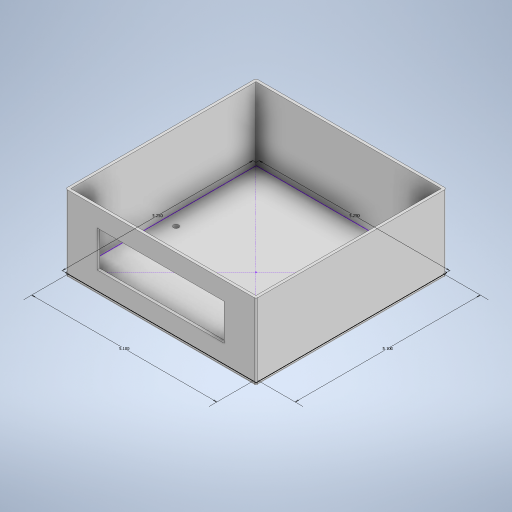
# Autodesk Inventor part: TC720 box
Saved by Autodesk Inventor 2024.1 (Build 281209000, 209)
## iProperties
Created: 2024-09-06
Part Number: TC720 box
Material: Generic
Document SubType Name: Modeling
Designer: pab2
Density: 1 g/cm^3
Appearance: Default
Author: pab2
Autodesk Inventor part; units mm, degrees
ref_plane "YZ Plane" through (0, 0, 0) normal (1, 0, 0) x (0, 1, 0)
ref_plane "XZ Plane" through (0, 0, 0) normal (0, 1, 0) x (-1, 0, 0)
ref_plane "XY Plane" through (0, 0, 0) normal (0, 0, 1) x (1, 0, 0)
sketch "Sketch1" plane through (0, 0, 0) normal (0, 1, 0) x (-1, 0, 0)
  line L0 (0, 0) -> (133.35, 0)
  line L1 (133.35, 0) -> (133.35, -133.35)
  line L2 (133.35, -133.35) -> (0, -133.35)
  line L3 (0, -133.35) -> (0, 0)
  line L4 (131.445, -131.445) -> (1.905, -131.445)
  line L5 (1.905, -131.445) -> (1.905, -1.905)
  line L6 (1.905, -1.905) -> (131.445, -1.905)
  line L7 (131.445, -1.905) -> (131.445, -131.445)
  line L8 (131.445, -131.445) -> (1.905, -1.905) construction
  line L9 (1.905, -131.445) -> (131.445, -1.905) construction
  point P0 (66.675, -66.675)
  dimension "d0" = 133.35
  dimension "d1" = 133.35
  dimension "d2" = 129.54
  dimension "d3" = 129.54
  constraints: 20 end point, 4 parallel, 2 horizontal, 2 midpoint, 2 perpendicular
  measures "d0" distance of L1.end L2.end
  measures "d1" distance of L0.end L1.end
  measures "d2" distance of L5.end L6.end
  measures "d3" distance of L4.end L5.end
extrude "Extrusion1" add sketch "Sketch1" along normal blind 50.8
extrude "Extrusion2" add sketch "Sketch1" against normal blind 2.54 contours L0 L1 L2 L3 | L4 L5 L6 L7
fillet "Fillet1" radius 1.27 8 edges at (0, 24.13, 0) (0, -2.54, -66.675) (-66.675, -2.54, 0) (0, 24.13, -133.35) (-66.675, -2.54, -133.35) (-133.35, 24.13, -133.35) (-133.35, -2.54, -66.675) (-133.35, 24.13, 0)
sketch "Sketch2" plane through (0, 0, 0) normal (0, 1, 0) x (1, 0, 0)
  line L0 (-131.445, 1.905) -> (-131.445, 131.445) projected
  line L1 (-1.905, 1.905) -> (-131.445, 1.905) projected
  line L2 (-1.905, 131.445) -> (-1.905, 1.905) projected
  line L3 (-131.445, 131.445) -> (-1.905, 131.445) projected
  line L4 (-66.675, 66.675) -> (-10.795, 66.675)
  line L5 (-66.675, 66.675) -> (-10.795, 66.675) construction
  line L6 (-10.795, 66.675) -> (-122.555, 66.675)
  point P0 (0, 0)
  dimension "d9" = 55.88
  dimension "d10" = 0
  dimension "d11" = 111.76
  constraints: 6 end point, 2 horizontal, 1 collinear, 1 point on line
  measures "d9" distance of L4.start L4.end
  measures "d10" distance between parallel lines of L4 L5
  measures "d11" distance of L4.end L6.end
hole "Hole1" at (-10.795, 0, -66.675) at (-122.555, 0, -66.675) direction (0, -1, 0) diameter 3.6576 end through all
sketch "Sketch3" plane through (-132.08, -1.27, 0) normal (0, 0, 1) x (1, 0, 0)
  line L0 (130.175, 1.27) -> (0.635, 1.27) projected
  line L1 (65.405, 1.27) -> (65.405, 13.97)
  line L2 (65.405, 13.97) -> (109.855, 13.97)
  line L3 (109.855, 13.97) -> (20.955, 13.97)
  line L4 (20.955, 13.97) -> (20.955, 39.37)
  line L5 (20.955, 39.37) -> (109.855, 39.37)
  line L6 (109.855, 39.37) -> (109.855, 13.97)
  point P0 (132.08, 1.27)
  dimension "d19" = 12.7
  dimension "d20" = 44.45
  dimension "d21" = 88.9
  dimension "d22" = 25.4
  constraints: 12 end point, 2 parallel, 2 perpendicular, 1 horizontal, 1 midpoint, 1 vertical
  measures "d19" distance of L1.start L1.end
  measures "d20" distance of L1.end L2.end
  measures "d21" distance of L4.end L5.end
  measures "d22" distance of L3.end L4.end
extrude "Extrusion3" cut sketch "Sketch3" against normal blind 2.54
body "Solid1"
